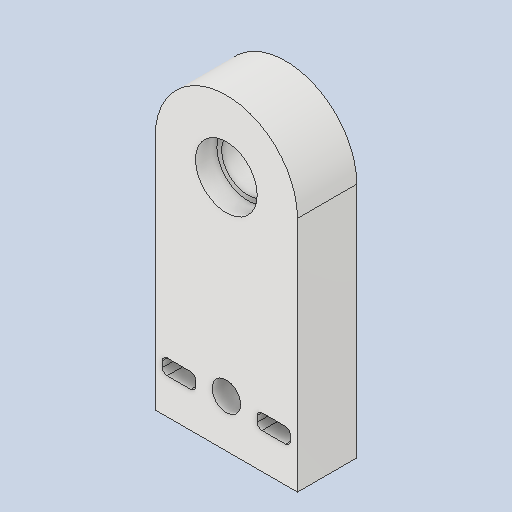
# Autodesk Inventor part: soporte_riel
Saved by Autodesk Inventor 2022 (Build 260153000, 153)
## iProperties
Created: 2019-06-12
Part Number: soporte_riel
Material: Nilón 6/6
Document SubType Name: Chapa
Designer: Usuario
Density: 1.13 g/cm^3
Appearance: Blanco
Sheet Metal Rule: Default
Author: Usuario
Autodesk Inventor part; units mm, degrees
ref_plane "YZ Plane" through (0, 0, 0) normal (1, 0, 0) x (0, 1, 0)
ref_plane "XZ Plane" through (0, 0, 0) normal (0, 1, 0) x (-1, 0, 0)
ref_plane "XY Plane" through (0, 0, 0) normal (0, 0, 1) x (1, 0, 0)
sketch "Boceto1" plane through (0, 0, 0) normal (0, 0, 1) x (1, 0, 0)
  point P0 (0, 0)
sketch "Boceto2" plane through (0, 0, 0) normal (0, 0, 1) x (1, 0, 0)
  line L0 (0, 0) -> (0, 100)
  line L1 (30, 130) -> (30, 130)
  line L2 (60, 100) -> (60, 0)
  line L3 (60, 0) -> (0, 0)
  arc A0 (30, 130) -> (0, 100) centre (30, 100) ccw
  arc A1 (60, 100) -> (30, 130) centre (30, 100) ccw
  point P0 (0, 130)
  point P1 (60, 130)
  dimension "d1" = 30
  dimension "d2" = 100
  dimension "d3" = 60
  constraints: 8 end point, 4 point on circle, 4 point on line, 4 tangent, 3 perpendicular, 2 centre point, 1 coincident, 1 concentric, 1 vertical
  measures "d1" radius of A0
  measures "d2" distance of L2.start L2.end
  measures "d3" distance of L2.end L0.start
extrude "Extrusión1" add sketch "Boceto2" along normal mid plane 25
sketch "Boceto9" plane through (0, 0, 12.5) normal (0, -1, 0) x (1, 0, 0)
  circle A0 centre (50, -12.5) radius 4
  line L0 (60, -25) -> (0, -25) projected
  circle A1 centre (10, -12.5) radius 4
  line L1 (0, -12.5) -> (60, -12.5) construction
  line L2 (60, 0) -> (60, -25) construction
  dimension "d52" = 8
  dimension "d88" = 10
  dimension "d89" = 10
  constraints: 2 centre point, 2 end point, 2 point on line, 1 equal radius, 1 horizontal
  measures "d52" diameter of A0
  measures "d88" distance of L1.start A1.centre
  measures "d89" distance from line of L2 A0.centre
hole "Agujero4" at (10, 0, 0) at (50, 0, 0) direction (0, 1, 0) diameter 8 depth 25
thread "Rosca3" size "M8x1.25" class "6H" standard "ANSI Metric M Profile" full length
thread "Rosca4" size "M8x1.25" class "6H" standard "ANSI Metric M Profile" full length
sketch "Boceto10" plane through (0, 0, 12.5) normal (0, 0, 1) x (1, 0, 0)
  circle A0 centre (30, 100) radius 11
  circle A1 centre (30, 100) radius 13.0125
  line L0 (60, 0) -> (60, 100) projected
  line L1 (0, 100) -> (0, 0) projected
  line L2 (40, 144.843) -> (20, 144.843) projected
  dimension "d64" = 22
  dimension "d65" = 30
  dimension "d68" = 26.025
  dimension "d90" = 100
  constraints: 2 centre point, 1 coincident
  measures "d64" diameter of A0
  measures "d65" distance from line of L0 A1.centre
  measures "d68" diameter of A1
  measures "d90" vertical distance of point (0, 0) A0.centre
extrude "Extrusión5" cut sketch "Boceto10" against normal through all contours A0
extrude "Extrusión6" cut sketch "Boceto10" against normal blind 9
sketch "Boceto12" plane through (0, 0, 12.5) normal (0, 0, 1) x (1, 0, 0)
  line L0 (5, 21.5) -> (15, 21.5)
  line L1 (17, 19.5) -> (17, 17)
  line L2 (15, 15) -> (5, 15)
  line L3 (3, 17) -> (3, 19.5)
  line L4 (45, 21.5) -> (55, 21.5)
  line L5 (57, 19.5) -> (57, 17)
  line L6 (55, 15) -> (45, 15)
  line L7 (43, 17) -> (43, 19.5)
  line L8 (0, 0) -> (60, 0) projected
  line L9 (10, 0) -> (10, 43.0314) construction
  line L10 (54, 0) -> (46, 0) construction
  line L11 (50, 0) -> (50, 39.0292) construction
  arc A0 (5, 21.5) -> (3, 19.5) centre (5, 19.5) ccw
  arc A1 (3, 17) -> (5, 15) centre (5, 17) ccw
  arc A2 (15, 15) -> (17, 17) centre (15, 17) ccw
  arc A3 (17, 19.5) -> (15, 21.5) centre (15, 19.5) ccw
  arc A4 (45, 21.5) -> (43, 19.5) centre (45, 19.5) ccw
  arc A5 (43, 17) -> (45, 15) centre (45, 17) ccw
  arc A6 (57, 19.5) -> (55, 21.5) centre (55, 19.5) ccw
  arc A7 (55, 15) -> (57, 17) centre (55, 17) ccw
  point P0 (17, 15)
  point P1 (17, 21.5)
  point P2 (3, 15)
  point P3 (43, 21.5)
  point P4 (57, 15)
  point P5 (43, 15)
  dimension "d91" = 14
  dimension "d92" = 14
  dimension "d93" = 6.5
  dimension "d94" = 15
  dimension "d95" = 40
  dimension "d96" = 7
  dimension "d97" = 7
  dimension "d98" = 2
  dimension "d99" = 2
  dimension "d100" = 2
  dimension "d101" = 2
  dimension "d102" = 2
  dimension "d103" = 2
  dimension "d104" = 2
  dimension "d105" = 2
  constraints: 20 end point, 16 point on circle, 16 tangent, 15 point on line, 8 centre point, 4 parallel, 2 horizontal, 2 perpendicular, 2 vertical, 1 midpoint
  measures "d91" distance of point (17, 15) point (3, 15)
  measures "d92" distance of point (57, 15) point (43, 15)
  measures "d93" distance of point (17, 21.5) point (17, 15)
  measures "d94" distance between parallel lines of L8 L2
  measures "d95" distance between parallel lines of L7 L3
  measures "d96" distance between parallel lines of L1 L9
  measures "d97" distance between parallel lines of L7 L11
  measures "d98" radius of A0
  measures "d99" radius of A1
  measures "d100" radius of A2
  measures "d101" radius of A3
  measures "d102" radius of A4
  measures "d103" radius of A5
  measures "d104" radius of A6
  measures "d105" radius of A7
extrude "Extrusión7" cut sketch "Boceto12" against normal blind 20
sketch "Boceto13" plane through (0, 0, 12.5) normal (0, 0, 1) x (1, 0, 0)
  circle A0 centre (30, 20) radius 6
  line L0 (0, 0) -> (60, 0) construction
  line L1 (30, 0) -> (30, 20) construction
  dimension "d108" = 20
  dimension "d109" = 12
  constraints: 2 end point, 1 centre point, 1 midpoint, 1 vertical
  measures "d108" vertical distance of L0.start L1.end
  measures "d109" diameter of A0
extrude "Extrusión8" cut sketch "Boceto13" against normal through all
equation "\"Radio_pliegue\" = Grosor"
equation "\"Anchura_desahogo_plegado\" = Grosor"
equation "\"Profundidad_desahogo_plegado\" = 0.5 * Grosor"
equation "\"Tamaño_destalonado\" = 4 * Grosor"
equation "\"Remanente_mínimo\" = 2 * Grosor"
equation "\"Radiodetransición\" = Radio_pliegue"
equation "\"Tamaño_de_radio_de_Jacobi\" = Grosor"
equation "\"TamañoSeparación\" = Grosor"
equation "\"Grosor\" = 0.5"
